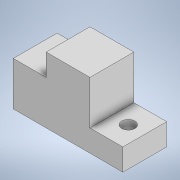
# Autodesk Inventor part: Peça3
Saved by Autodesk Inventor 2021 (Build 250183000, 183)
## iProperties
Created: 2022-02-08
Part Number: Peça3
Material: Genérico
Document SubType Name: Modeling
Designer: aluno
Density: 1 g/cm^3
Appearance: Padrão
Author: aluno
Autodesk Inventor part; units mm, degrees
ref_plane "YZ Plane" through (0, 0, 0) normal (1, 0, 0) x (0, 1, 0)
ref_plane "XZ Plane" through (0, 0, 0) normal (0, 1, 0) x (-1, 0, 0)
ref_plane "XY Plane" through (0, 0, 0) normal (0, 0, 1) x (1, 0, 0)
sketch "Esboço1" plane through (0, 0, 0) normal (0, 0, 1) x (1, 0, 0)
  line L0 (0, 0) -> (50, 0)
  line L1 (50, 0) -> (50, 10)
  line L2 (0, 0) -> (0, 20)
  line L3 (0, 20) -> (15, 20)
  line L4 (15, 20) -> (15, 30)
  line L5 (15, 30) -> (35, 30)
  line L6 (35, 30) -> (35, 10)
  line L7 (35, 10) -> (50, 10)
  dimension "d0" = 50
  dimension "d1" = 10
  dimension "d2" = 20
  dimension "d3" = 15
  dimension "d4" = 10
  dimension "d5" = 20
  constraints: 16 end point, 6 perpendicular, 1 horizontal, 1 vertical
  measures "d0" distance of L0.start L0.end
  measures "d1" distance of L0.end L1.end
  measures "d2" distance of L0.start L2.end
  measures "d3" distance of L2.end L3.end
  measures "d4" distance of L3.end L4.end
  measures "d5" distance of L4.end L5.end
extrude "Extrusão1" add sketch "Esboço1" along normal blind 20
sketch "Esboço2" plane through (35, 10, 0) normal (0, 1, 0) x (1, 0, 0)
  line L0 (15, 0) -> (15, -20) projected
  line L1 (15, -20) -> (0, -20) projected
  point P0 (-35, 0)
  point P1 (7.5, -10)
  dimension "d8" = 7.5
  dimension "d16" = 10
  measures "d8" distance from line of L0 point (7.5, -10)
  measures "d16" distance from line of L1 point (7.5, -10)
hole "Furo1" at (42.5, 10, 10) direction (0, -1, 0) diameter 6 end through all
